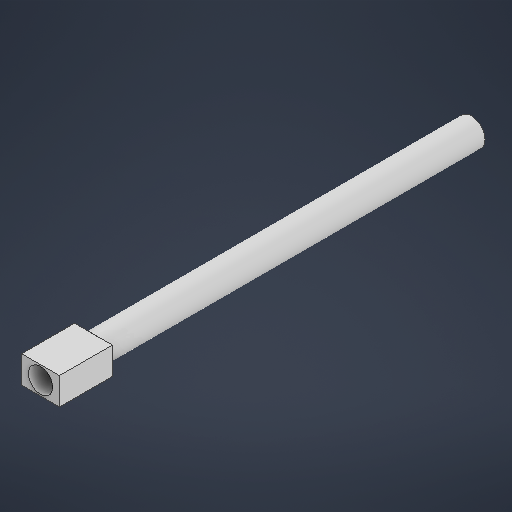
# Autodesk Inventor part: motor_arm
Saved by Autodesk Inventor 2026.1 (Build 301233000, 233)
## iProperties
Created: 2025-09-08
Part Number: motor_arm
Material: 일반
Document SubType Name: Modeling
Designer: ytw32
Density: 1 g/cm^3
Appearance: 기본값
Author: ytw32
Autodesk Inventor part; units mm, degrees
ref_plane "YZ Plane" through (0, 0, 0) normal (1, 0, 0) x (0, 1, 0)
ref_plane "XZ Plane" through (0, 0, 0) normal (0, 1, 0) x (-1, 0, 0)
ref_plane "XY Plane" through (0, 0, 0) normal (0, 0, 1) x (1, 0, 0)
sketch "스케치1" plane through (0, 0, 0) normal (0, 0, 1) x (1, 0, 0)
  circle A0 centre (0, 0) radius 18
  circle A1 centre (0, 0) radius 16
  dimension "d0" = 36
  dimension "d1" = 32
  constraints: 2 centre point, 2 coincident
  measures "d0" diameter of A0
  measures "d1" diameter of A1
extrude "돌출1" add sketch "스케치1" along normal mid plane 500
sketch "스케치2" plane through (0, 0, 250) normal (0, 0, 1) x (1, 0, 0)
  line L0 (-25, 18) -> (25, 18)
  line L1 (25, 18) -> (25, -18)
  line L2 (25, -18) -> (-25, -18)
  line L3 (-25, -18) -> (-25, 18)
  line L4 (-25, 18) -> (25, -18) construction
  line L5 (25, 18) -> (-25, -18) construction
  point P0 (0, 0)
  dimension "d4" = 50
  constraints: 12 end point, 2 midpoint, 2 parallel, 1 horizontal, 1 perpendicular
  measures "d4" distance of L1.end L2.end
extrude "돌출2" add sketch "스케치2" along normal blind 70
sketch "스케치3" plane through (0, 0, 320) normal (0, 0, 1) x (1, 0, 0)
  circle A0 centre (0, 0) radius 16
  constraints: 1 centre point, 1 coincident
extrude "돌출3" cut sketch "스케치3" against normal blind 70
